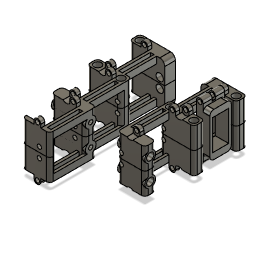
engine block (Autodesk Fusion 360 design; units mm, degrees)
Autodesk Fusion 360 part; units mm, degrees
note: some values were not read from the file. Chosen so that the rebuilt part matches the saved one: which face or edge a step refers to; which sketch regions a step uses.
sketch "Sketch1" plane through (0, 0, 0) normal (0, 1, 0) x (1, 0, 0)
  line L0 (0, 0) -> (2.7, 0)
  line L1 (2.7, 0) -> (2.7, -23.6)
  line L2 (2.7, -23.6) -> (0, -23.6)
  line L3 (0, -23.6) -> (0, 0)
  line L4 (-2, 2) -> (4.7, 2)
  line L5 (4.7, 2) -> (4.7, -25.6)
  line L6 (4.7, -25.6) -> (-2, -25.6)
  line L7 (-2, -25.6) -> (-2, 2)
  dimension "d1" = 2.7
  dimension "d2" = 23.6
  dimension "d3" = 2
  dimension "d4" = 2
  dimension "d5" = 2
  dimension "d6" = 2
  constraint horizontal L0
  constraint vertical L1
  constraint horizontal L2
  constraint vertical L3
  constraint coincident L0.start L3.end
  constraint horizontal L4
  constraint vertical L5
  constraint horizontal L6
  constraint vertical L7
  measures "d1" distance of L0.start L0.end
  measures "d2" distance of L0.start L2.end
  measures "d3" distance of L0 L4
  measures "d4" distance of L1 L5
  measures "d5" distance of L3 L7
  measures "d6" distance of L2 L6
extrude "Extrude1" add sketch "Sketch1" along normal blind 5 makes body 1
sketch "Sketch2" plane through (0, 5, 0) normal (0, 1, 0) x (-1, 0, 0)
  line L0 (-2.7, 23.6) -> (0, 23.6)
  line L1 (0, 23.6) -> (0, 0)
  line L2 (0, 0) -> (-2.7, 0)
  line L3 (-2.7, 0) -> (-2.7, 23.6)
  line L4 (2, 25.6) -> (-4.7, 25.6)
  line L5 (-4.7, 25.6) -> (-4.7, -2)
  line L6 (-4.7, -2) -> (2, -2)
  line L7 (2, -2) -> (2, 25.6)
  line L8 (2, -2) -> (-18.4, -2)
  line L9 (-18.4, -2) -> (-18.4, 0)
  line L10 (-18.4, 0) -> (2, 0)
  line L11 (2, 0) -> (2, -2)
  line L12 (2, 25.6) -> (-18.4, 25.6)
  line L13 (-18.4, 25.6) -> (-18.4, 23.6)
  line L14 (-18.4, 23.6) -> (2, 23.6)
  line L15 (2, 23.6) -> (2, 25.6)
  dimension "d9" = 20.4
  dimension "d10" = 20.4
  constraint horizontal L8
  constraint vertical L9
  constraint horizontal L10
  constraint vertical L11
  constraint coincident L6.end L7.start
  constraint coincident L1.end L10
  constraint horizontal L12
  constraint vertical L13
  constraint horizontal L14
  constraint vertical L15
  constraint coincident L4.start L7.end
  constraint coincident L0.end L14
  measures "d9" distance of L6.end L8.end
  measures "d10" distance of L4.start L12.end
extrude "Extrude2" add sketch "Sketch2" along normal blind 11.25 and the other way blind 5 contours L0 L4 L5 L7 L12 L14 L15 | L2 L5 L6 L7 L8 L10 L11 | L5 L12 L13 L14 | L5 L8 L9 L10 bodies 1
copy_body "CopyPasteBodies1" bodies 1 makes body 2
move_body "Move1" bodies 2 to x (1, 0, 0) y (0, 1, 0) z (0, 0, 1) at (-5, 0, 31.6)
extrude "Extrude3" add 1 faces at (-0.2, 5.4167, 29.6) along direction (0, 0, -1) blind 4 on bodies 2 bodies 2 1
extrude "Extrude4" add 1 faces at (-5.3333, 5.4167, 25.6) along direction (0, 0, -1) blind 2 on bodies 2 bodies 2
extrude "Extrude5" add 1 faces at (13.4, 5.4167, 27.6) along direction (1, 0, 0) blind 5 on bodies 2 bodies 2
sketch "Sketch3" plane through (0, 0, 0) normal (0, -1, 0) x (1, 0, 0)
  line L0 (2.7, 0) -> (0, 0)
  line L1 (0, 0) -> (0, 23.6)
  line L2 (0, 23.6) -> (2.7, 23.6)
  line L3 (2.7, 23.6) -> (2.7, 0)
  line L4 (-0.3, 31.6) -> (-0.3, 55.2)
  line L5 (-0.3, 55.2) -> (13.4, 55.2)
  line L6 (13.4, 55.2) -> (13.4, 57.2)
  line L7 (13.4, 57.2) -> (-7, 57.2)
  line L8 (-7, 57.2) -> (-7, 23.6)
  line L9 (-7, 23.6) -> (-2, 23.6)
  line L10 (-2, 23.6) -> (-2, -2)
  line L11 (-2, -2) -> (18.4, -2)
  line L12 (18.4, -2) -> (18.4, 0)
  line L13 (18.4, 0) -> (4.7, 0)
  line L14 (4.7, 0) -> (4.7, 23.6)
  line L15 (4.7, 23.6) -> (18.4, 23.6)
  line L16 (18.4, 23.6) -> (18.4, 31.6)
  line L17 (18.4, 31.6) -> (-0.3, 31.6)
  line L18 (-2.3, 31.6) -> (-5, 31.6)
  line L19 (-5, 31.6) -> (-5, 55.2)
  line L20 (-5, 55.2) -> (-2.3, 55.2)
  line L21 (-2.3, 55.2) -> (-2.3, 31.6)
  line L22 (-7, 23.6) -> (1, 23.6) construction
  line L23 (1, 23.6) -> (1, 31.6) construction
  line L24 (1, 31.6) -> (-7, 31.6) construction
  line L25 (-7, 31.6) -> (-7, 23.6) construction
  line L26 (-7, 31.6) -> (1, 23.6) construction
  circle A0 centre (-3, 27.6) radius 1.65
  circle A1 centre (-3, 27.6) radius 2.75
  line L27 (18.4, 31.6) -> (10.4, 31.6) construction
  line L28 (10.4, 31.6) -> (10.4, 23.6) construction
  line L29 (10.4, 23.6) -> (18.4, 23.6) construction
  line L30 (18.4, 23.6) -> (18.4, 31.6) construction
  line L31 (18.4, 31.6) -> (10.4, 23.6) construction
  circle A2 centre (14.4, 27.6) radius 1.65
  circle A3 centre (14.4, 27.6) radius 2.75
  dimension "d21" = 8
  dimension "d22" = 8
  dimension "d23" = 3.3
  dimension "d24" = 5.5
  dimension "d28" = 8
  dimension "d29" = 3.3
  dimension "d30" = 5.5
  constraint horizontal L22
  constraint vertical L23
  constraint horizontal L24
  constraint vertical L25
  constraint coincident L8.end L9.start
  constraint midpoint L26 A0.centre
  constraint concentric A0 A1
  constraint horizontal L27
  constraint vertical L28
  constraint horizontal L29
  constraint vertical L30
  constraint coincident L15 L28.end
  constraint coincident L16.end L17.start
  constraint midpoint L31 A2.centre
  constraint concentric A2 A3
  measures "d21" distance of L8.end L22.end
  measures "d22" distance of L8.end L24.end
  measures "d23" diameter of A0
  measures "d24" diameter of A1
  measures "d28" distance of L16.end L27.end
  measures "d29" diameter of A2
  measures "d30" diameter of A3
extrude "Extrude6" cut sketch "Sketch3" against normal through all contours A0 | A2 bodies 2
extrude "Extrude7" cut sketch "Sketch3" against normal blind 5 contours A1 | A3 bodies 2
fillet "Fillet1" radius 2.5 4 edges at (18.4, 8.125, 23.6) (18.4, 8.125, 31.6) (-7, 10.625, 31.6) (-7, 8.125, 23.6) on bodies 2
extrude "Extrude8" add 1 faces at (6.6, 5.4167, 57.2) along direction (0, 0, 1) blind 6 on bodies 2 bodies 2
fillet "Fillet2" radius 2.5 4 edges at (13.4, 8.125, 63.2) (13.4, 8.125, 55.2) (-7, 10.625, 55.2) (-7, 8.125, 63.2) on bodies 2
sketch "Sketch4" plane through (0, 0, 63.2) normal (0, 0, 1) x (1, 0, 0)
  line L0 (-4.5, 16.25) -> (-4.5, 0)
  line L1 (-4.5, 0) -> (10.9, 0)
  line L2 (10.9, 0) -> (10.9, 16.25)
  line L3 (10.9, 16.25) -> (-4.5, 16.25)
  line L4 (13.4, 0) -> (13.4, 16.25) construction
  line L5 (-0.3, 0) -> (13.4, 0) construction
  line L6 (-0.3, -5) -> (4.7, -5) construction
  line L7 (4.7, -5) -> (4.7, 0) construction
  line L8 (4.7, 0) -> (-0.3, 0) construction
  line L9 (-0.3, 0) -> (-0.3, -5) construction
  line L10 (4.7, 0) -> (-0.3, -5) construction
  arc A0 (-0.3, -2.5) -> (4.7, -2.5) centre (2.2, -2.5) ccw
  line L11 (-0.3, 0) -> (-0.3, -2.5)
  line L12 (4.7, -2.5) -> (4.7, 0)
  circle A1 centre (2.2, -2.5) radius 1.6
  point P0 (-0.3, 0)
  dimension "d38" = 5
  dimension "d39" = 5
  dimension "d40" = 3.2
  constraint coincident P0 L5.start
  constraint coincident L4.start L5.end
  constraint horizontal L6
  constraint vertical L7
  constraint horizontal L8
  constraint vertical L9
  constraint midpoint L7 A0.end
  constraint midpoint L9 A0.start
  constraint midpoint L10 A0.centre
  constraint concentric A0 A1
  measures "d38" distance of L6.start L6.end
  measures "d39" distance of L6.start P0
  measures "d40" diameter of A1
extrude "Extrude9" add sketch "Sketch4" against normal blind 3 from surface at -5 contours L1 A0 L11 L12 bodies 2
extrude "Extrude10" add sketch "Sketch4" against normal blind 3 from surface at -31.6 contours L1 A0 L11 L12 bodies 2
sketch "Sketch5" plane through (0, 0, 23.6) normal (0, 0, -1) x (-1, 0, 0)
  line L0 (4.5, 0) -> (4.5, 16.25)
  line L1 (4.5, 16.25) -> (-15.9, 16.25)
  line L2 (-15.9, 16.25) -> (-15.9, 0)
  line L3 (-15.9, 0) -> (-4.7, 0)
  line L4 (-4.7, 0) -> (-4.7, 5)
  line L5 (-4.7, 5) -> (-2.7, 5)
  line L6 (-2.7, 5) -> (-2.7, 0)
  line L7 (-2.7, 0) -> (0, 0)
  line L8 (0, 0) -> (0, 5)
  line L9 (0, 5) -> (2, 5)
  line L10 (2, 5) -> (2, 0)
  line L11 (2, 0) -> (4.5, 0)
  line L12 (-4.7, 0) -> (-9.7, 0) construction
  line L13 (-9.7, 0) -> (-9.7, -5) construction
  line L14 (-9.7, -5) -> (-4.7, -5) construction
  line L15 (-4.7, -5) -> (-4.7, 0) construction
  line L16 (-4.7, 0) -> (-9.7, -5) construction
  arc A0 (-9.7, -2.5) -> (-4.7, -2.5) centre (-7.2, -2.5) ccw
  line L17 (-9.7, 0) -> (-9.7, -2.5)
  line L18 (-4.7, -2.5) -> (-4.7, 0)
  circle A1 centre (-7.2, -2.5) radius 1.6
  dimension "d47" = 5
  dimension "d48" = 5
  dimension "d49" = 3.2
  constraint horizontal L12
  constraint vertical L13
  constraint horizontal L14
  constraint vertical L15
  constraint coincident L3.end L4.start
  constraint midpoint L15 A0.end
  constraint midpoint L16 A0.centre
  constraint tangent A0 L17
  constraint concentric A0 A1
  measures "d47" distance of L3.end L12.end
  measures "d48" distance of L3.end L14.end
  measures "d49" diameter of A1
extrude "Extrude11" add sketch "Sketch5" against normal blind 3 contours L3 A0 L17 L18 bodies 2
extrude "Extrude12" add sketch "Sketch5" along normal blind 3 from surface at 23.6 contours L3 A0 L17 L18 bodies 2
extrude "Extrude13" add 1 faces at (8.7, 10.8333, -2) along direction (0, 0, -1) blind 6 on bodies 2 bodies 2
fillet "Fillet3" radius 2.5 2 edges at (18.4, 8.125, 0) (18.4, 8.125, -8) on bodies 2
sketch "Sketch7" plane through (-2, 0, 0) normal (-1, 0, 0) x (0, 0, 1)
  line L0 (23.6, 0) -> (23.6, 5)
  line L1 (23.6, 5) -> (0, 5)
  line L2 (0, 5) -> (0, 16.25)
  line L3 (0, 16.25) -> (-8, 16.25)
  line L4 (-8, 16.25) -> (-8, 0)
  line L5 (-8, 0) -> (23.6, 0)
  line L6 (0, 5) -> (0, 0)
  constraint coincident L1.end L2.start
  constraint coincident L6.end origin
extrude "Extrude16" add sketch "Sketch7" along normal blind 6 contours L2 L3 L4 L5 L6 bodies 2
sketch "Sketch8" plane through (0, 0, 0) normal (0, 0, 1) x (1, 0, 0)
  line L0 (15.9, 0) -> (15.9, 16.25)
  line L1 (15.9, 16.25) -> (-8, 16.25)
  line L2 (-8, 16.25) -> (-8, 0)
  line L3 (-8, 0) -> (-2, 0)
  line L4 (-2, 0) -> (-2, 5)
  line L5 (-2, 5) -> (0, 5)
  line L6 (0, 5) -> (0, 0)
  line L7 (0, 0) -> (2.7, 0)
  line L8 (2.7, 0) -> (2.7, 5)
  line L9 (2.7, 5) -> (4.7, 5)
  line L10 (4.7, 5) -> (4.7, 0)
  line L11 (4.7, 0) -> (4.7, -2.5)
  arc A0 (4.7, -2.5) -> (9.7, -2.5) centre (7.2, -2.5) ccw
  line L12 (9.7, -2.5) -> (9.7, 0)
  line L13 (9.7, 0) -> (15.9, 0)
  circle A1 centre (7.2, -2.5) radius 1.6
  circle A2 centre (-4.25, 12.5) radius 3.75
  circle A3 centre (-4.25, 12.5) radius 2.75
  circle A4 centre (-4.25, 12.5) radius 1.6
  circle A5 centre (-4.25, 3.75) radius 3.75
  dimension "d69" = 5.5
  dimension "d70" = 1
  dimension "d71" = 3.2
  constraint tangent L2 A2
  constraint tangent L1 A2
  constraint concentric A2 A3
  constraint concentric A2 A4
  constraint tangent L3 A5
  constraint tangent L2 A5
  constraint equal A2 A5
  measures "d69" diameter of A3
  measures "d70" distance of A2 A3
  measures "d71" diameter of A4
extrude "Extrude17" cut sketch "Sketch8" against normal through all contours L2 L3 A5 | A4 bodies 2
extrude "Extrude18" cut sketch "Sketch8" against normal blind 4 contours A3 bodies 2
sketch "Sketch9" plane through (13.4, 0, 0) normal (1, 0, 0) x (0, 0, -1)
  line L0 (-57.7, 0) -> (-57.7, 16.25)
  line L1 (-57.7, 16.25) -> (-60.7, 16.25)
  line L2 (-60.7, 16.25) -> (-60.7, 0)
  line L3 (-60.7, 0) -> (-57.7, 0)
  line L4 (-60.7, 16.25) -> (-57.7, 0) construction
  circle A0 centre (-59.2, 8.125) radius 1.6
  line L5 (-55.2, 0) -> (-55.2, 16.25)
  line L6 (-63.2, 16.25) -> (-63.2, 0)
  circle A1 centre (-59.2, 8.125) radius 4
  circle A2 centre (-59.2, 8.125) radius 2.75
  dimension "d75" = 3.2
  dimension "d79" = 5.5
  constraint coincident L1.end L2.start
  constraint coincident L0.start L3.end
  constraint midpoint L4 A0.centre
  constraint concentric A0 A1
  constraint tangent L5 A1
  constraint concentric A0 A2
  measures "d75" diameter of A0
  measures "d79" diameter of A2
extrude "Extrude19" add sketch "Sketch9" against normal up to surface (20.4 mm away) contours L0 L2 A1 A2 | L0 A1 A2 | L0 L2 A0 A2 | L0 A0 A2 | L2 A1 A2 | L2 A0 A2 | L0 L2 A1 A2 | L0 L2 A0 A2 bodies 2
extrude "Extrude20" cut sketch "Sketch9" against normal through all contours L0 L2 A0 | L0 A0 | L2 A0 bodies 2
extrude "Extrude21" cut sketch "Sketch9" against normal blind 16 contours L0 L2 A0 A2 | L0 A0 A2 | L2 A0 A2 | L0 L2 A0 A2 bodies 2
extrude "Extrude22" cut sketch "Sketch8" along normal through all contours A4 bodies 2
sketch "Sketch20" plane through (0, 0, 0) normal (0, -1, 0) x (1, 0, 0)
  line L0 (-4.25, 0) -> (-4.25, -8)
  line L1 (-4.25, -8) -> (15.9, -8)
  arc A0 (15.9, -8) -> (18.4, -5.5) centre (15.9, -5.5) ccw
  line L2 (18.4, -5.5) -> (18.4, -2.5)
  arc A1 (18.4, -2.5) -> (15.9, 0) centre (15.9, -2.5) ccw
  line L3 (15.9, 0) -> (9.7, 0)
  line L4 (9.7, 0) -> (9.7, -3)
  line L5 (9.7, -3) -> (4.7, -3)
  line L6 (4.7, -3) -> (4.7, 0)
  line L7 (4.7, 0) -> (4.7, 23.6)
  line L8 (4.7, 23.6) -> (4.7, 26.6)
  line L9 (4.7, 26.6) -> (9.7, 26.6)
  line L10 (9.7, 26.6) -> (9.7, 23.6)
  line L11 (9.7, 23.6) -> (15.9, 23.6)
  arc A2 (15.9, 23.6) -> (18.4, 26.1) centre (15.9, 26.1) ccw
  line L12 (18.4, 26.1) -> (18.4, 29.1)
  arc A3 (18.4, 29.1) -> (15.9, 31.6) centre (15.9, 29.1) ccw
  line L13 (15.9, 31.6) -> (4.7, 31.6)
  line L14 (4.7, 31.6) -> (4.7, 28.6)
  line L15 (4.7, 28.6) -> (-0.3, 28.6)
  line L16 (-0.3, 28.6) -> (-0.3, 31.6)
  line L17 (-0.3, 31.6) -> (-0.3, 55.2)
  line L18 (-0.3, 55.2) -> (-0.3, 58.2)
  line L19 (-0.3, 58.2) -> (4.7, 58.2)
  line L20 (4.7, 58.2) -> (4.7, 55.2)
  line L21 (4.7, 55.2) -> (10.9, 55.2)
  arc A4 (10.9, 55.2) -> (13.4, 57.7) centre (10.9, 57.7) ccw
  line L22 (13.4, 57.7) -> (13.4, 60.7)
  arc A5 (13.4, 60.7) -> (10.9, 63.2) centre (10.9, 60.7) ccw
  line L23 (10.9, 63.2) -> (-4.5, 63.2)
  arc A6 (-4.5, 63.2) -> (-7, 60.7) centre (-4.5, 60.7) ccw
  line L24 (-7, 60.7) -> (-7, 26.1)
  arc A7 (-7, 26.1) -> (-4.5, 23.6) centre (-4.5, 26.1) ccw
  line L25 (-4.5, 23.6) -> (-2, 23.6)
  line L26 (-2, 23.6) -> (-2, 0)
  line L27 (-2, 0) -> (-4.25, 0)
  line L28 (2.7, 0) -> (0, 0)
  line L29 (0, 0) -> (0, 23.6)
  line L30 (0, 23.6) -> (2.7, 23.6)
  line L31 (2.7, 23.6) -> (2.7, 0)
  circle A8 centre (14.4, 27.6) radius 2.75
  circle A9 centre (-3, 27.6) radius 2.75
  line L32 (-5, 31.5495) -> (-5, 55.2505)
  arc A10 (-5, 55.2505) -> (-4.5, 55.2) centre (-4.5, 57.7) ccw
  line L33 (-4.5, 55.2) -> (-2.3, 55.2)
  line L34 (-2.3, 55.2) -> (-2.3, 31.6)
  line L35 (-2.3, 31.6) -> (-4.5, 31.6)
  arc A11 (-4.5, 31.6) -> (-5, 31.5495) centre (-4.5, 29.1) ccw
  circle A12 centre (14.4, -4) radius 4 construction
  circle A13 centre (14.4, -4) radius 1.6
  circle A14 centre (14.4, -4) radius 2.75
  dimension "d179" = 3.2
  dimension "d180" = 5.5
  constraint tangent L3 A12
  constraint tangent L2 A12
  constraint tangent L1 A12
  constraint concentric A12 A13
  constraint concentric A12 A14
  measures "d179" diameter of A13
  measures "d180" diameter of A14
extrude "Extrude41" cut sketch "Sketch20" against normal through all contours A13 bodies 2
extrude "Extrude42" cut sketch "Sketch20" against normal blind 5 contours A14 bodies 2
mirror "Mirror3" about plane through (-8, 0, 0) normal (-1, 0, 0) of bodies 2 makes body 3
move_body "Move2" bodies 3 to x (1, 0, 0) y (0, 1, 0) z (0, 0, 1) at (-20, 0, 0)
delete_face "DeleteFace1" 6 faces at (-30.7381, 4.7496, 63.0811) (-31.2766, 4.375, 55.21) (-30.4908, 8.3436, 55.206) (-31.2495, 9.2965, 55.2126) (-30.0678, 10.8018, 62.7491) (-30.1428, 7.2575, 63.1048) on bodies 3
sketch "Sketch12" plane through (0, 0, 0) normal (0, -1, 0) x (1, 0, 0)
  line L0 (-31, 55.2) -> (-31, 31.5495)
  arc A0 (-31, 31.5495) -> (-31.5, 31.6) centre (-31.5, 29.1) ccw
  line L1 (-31.5, 31.6) -> (-33.7, 31.6)
  line L2 (-33.7, 31.6) -> (-33.7, 55.2)
  line L3 (-33.7, 55.2) -> (-31, 55.2)
  circle A1 centre (-33, 27.6) radius 2.75
  circle A2 centre (-50.4, 27.6) radius 2.75
  line L4 (-36, 0) -> (-38.7, 0)
  line L5 (-38.7, 0) -> (-38.7, 23.6)
  line L6 (-38.7, 23.6) -> (-36, 23.6)
  line L7 (-36, 23.6) -> (-36, 0)
  line L8 (-29, 26.1) -> (-29, 63.2)
  line L9 (-29, 63.2) -> (-46.9, 63.2)
  arc A3 (-46.9, 63.2) -> (-49.4, 60.7) centre (-46.9, 60.7) ccw
  line L10 (-49.4, 60.7) -> (-49.4, 57.7)
  arc A4 (-49.4, 57.7) -> (-46.9, 55.2) centre (-46.9, 57.7) ccw
  line L11 (-46.9, 55.2) -> (-40.7, 55.2)
  line L12 (-40.7, 55.2) -> (-40.7, 58.2)
  line L13 (-40.7, 58.2) -> (-35.7, 58.2)
  line L14 (-35.7, 58.2) -> (-35.7, 55.2)
  line L15 (-35.7, 55.2) -> (-35.7, 31.6)
  line L16 (-35.7, 31.6) -> (-35.7, 28.6)
  line L17 (-35.7, 28.6) -> (-40.7, 28.6)
  line L18 (-40.7, 28.6) -> (-40.7, 31.6)
  line L19 (-40.7, 31.6) -> (-51.9, 31.6)
  arc A5 (-51.9, 31.6) -> (-54.4, 29.1) centre (-51.9, 29.1) ccw
  line L20 (-54.4, 29.1) -> (-54.4, 26.1)
  arc A6 (-54.4, 26.1) -> (-51.9, 23.6) centre (-51.9, 26.1) ccw
  line L21 (-51.9, 23.6) -> (-45.7, 23.6)
  line L22 (-45.7, 23.6) -> (-45.7, 26.6)
  line L23 (-45.7, 26.6) -> (-40.7, 26.6)
  line L24 (-40.7, 26.6) -> (-40.7, 23.6)
  line L25 (-40.7, 23.6) -> (-40.7, 0)
  line L26 (-40.7, 0) -> (-40.7, -3)
  line L27 (-40.7, -3) -> (-45.7, -3)
  line L28 (-45.7, -3) -> (-45.7, 0)
  line L29 (-45.7, 0) -> (-51.9, 0)
  arc A7 (-51.9, 0) -> (-54.4, -2.5) centre (-51.9, -2.5) ccw
  line L30 (-54.4, -2.5) -> (-54.4, -5.5)
  arc A8 (-54.4, -5.5) -> (-51.9, -8) centre (-51.9, -5.5) ccw
  line L31 (-51.9, -8) -> (-31.75, -8)
  line L32 (-31.75, -8) -> (-31.75, 0)
  line L33 (-31.75, 0) -> (-34, 0)
  line L34 (-34, 0) -> (-34, 23.6)
  line L35 (-34, 23.6) -> (-31.5, 23.6)
  arc A9 (-31.5, 23.6) -> (-29, 26.1) centre (-31.5, 26.1) ccw
  line L36 (-33.7, 55.2) -> (-33.7, 63.2) construction
  line L37 (-33.7, 63.2) -> (-28.7, 63.2) construction
  line L38 (-28.7, 63.2) -> (-26, 63.2)
  line L39 (-26, 63.2) -> (-26, 86.8)
  line L40 (-26, 86.8) -> (-28.7, 86.8)
  line L41 (-28.7, 86.8) -> (-28.7, 63.2)
  line L42 (-24, 88.8) -> (-30.7, 88.8)
  line L43 (-30.7, 88.8) -> (-30.7, 61.2)
  line L44 (-30.7, 61.2) -> (-24, 61.2) construction
  line L45 (-24, 61.2) -> (-24, 88.8)
  line L46 (-31, 55.2) -> (-24, 55.2)
  line L47 (-24, 55.2) -> (-24, 61.2)
  line L48 (-24, 61.2) -> (-31, 61.2)
  line L49 (-31, 61.2) -> (-31, 55.2) construction
  line L50 (-24, 86.8) -> (-44.4, 86.8) construction
  line L51 (-44.4, 86.8) -> (-44.4, 89.8)
  line L52 (-44.4, 89.8) -> (-24, 89.8)
  line L53 (-24, 89.8) -> (-24, 86.8)
  line L54 (-30.7, 86.8) -> (-44.4, 86.8)
  circle A10 centre (-50.4, -4) radius 2.75
  dimension "d107" = 5
  dimension "d108" = 2.7
  dimension "d109" = 23.6
  dimension "d110" = 2
  dimension "d111" = 2
  dimension "d112" = 2
  dimension "d113" = 2
  dimension "d114" = 20.4
  dimension "d115" = 3
  constraint coincident L2.end L3.start
  constraint coincident L9 L36.end
  constraint perpendicular L9 L36
  constraint perpendicular L36 L37
  constraint horizontal L38
  constraint vertical L39
  constraint horizontal L40
  constraint vertical L41
  constraint horizontal L42
  constraint vertical L43
  constraint horizontal L44
  constraint vertical L45
  constraint horizontal L46
  constraint vertical L47
  constraint horizontal L48
  constraint vertical L49
  constraint coincident L0.start L3.end
  constraint horizontal L50
  constraint vertical L51
  constraint horizontal L52
  constraint vertical L53
  constraint coincident L45 L50.start
  constraint coincident L39.end L50
  constraint coincident L50 L54.start
  constraint coincident L43 L54.start
  measures "d107" distance of L36.end L37.end
  measures "d108" distance of L37.end L38.end
  measures "d109" distance of L37.end L40.end
  measures "d110" distance of L40 L42
  measures "d111" distance of L39 L45
  measures "d112" distance of L41 L43
  measures "d113" distance of L38 L44
  measures "d114" distance of L50.start L50.end
  measures "d115" distance of L50.start L52.end
extrude "Extrude26" add sketch "Sketch12" against normal blind 5 contours L8 L9 L42 L43 L45 L48 L53 bodies 3
extrude "Extrude27" add sketch "Sketch12" against normal up to surface (16.25 mm away) contours L8 L46 L47 L48 | L42 L43 L51 L52 L53 L54 bodies 3
extrude "Extrude29" cut 1 faces at (-29, 8.5869, 59.1707) along direction (1, 0, 0) blind 5 on bodies 3 bodies 3
extrude "Extrude28" add 1 faces at (-29, 12.5, 61.8667) along direction (1, 0, 0) blind 5 on bodies 3 bodies 3
extrude "Extrude36" add 1 faces at (-26.2333, 8.75, 88.8) along direction (0, 0, -1) blind 2 on bodies 3 bodies 3
fillet "Fillet5" radius 2.5 4 edges at (-24, 10.625, 63.2) (-24, 8.125, 55.2) (-24, 8.125, 89.8) (-44.4, 8.125, 89.8) on bodies 3
extrude "Extrude30" add 1 faces at (-33.4, 6.016, 60.2599) along direction (-1, 0, 0) blind 2 from surface at -9.4 on bodies 3 bodies 3
extrude "Extrude31" add 1 faces at (-49.4, 2.9446, 59.7) along direction (-1, 0, 0) blind 7 from surface at -25.4 on bodies 3 bodies 3
sketch "Sketch13" plane through (0, 0, 63.2) normal (0, 0, 1) x (1, 0, 0)
  line L0 (-26.5, 8.125) -> (-26.5, 16.25)
  line L1 (-26.5, 16.25) -> (-46.9, 16.25)
  line L2 (-46.9, 16.25) -> (-46.9, 8.125)
  line L3 (-46.9, 8.125) -> (-46.9, 0)
  line L4 (-46.9, 0) -> (-30.7, 0)
  line L5 (-30.7, 0) -> (-30.7, 5)
  line L6 (-30.7, 5) -> (-28.7, 5)
  line L7 (-28.7, 5) -> (-28.7, 0)
  line L8 (-28.7, 0) -> (-26.5, 0)
  line L9 (-26.5, 0) -> (-26.5, 8.125)
  circle A0 centre (-31.75, 12.5) radius 1.6
extrude "Extrude32" cut sketch "Sketch13" along normal blind -8 and the other way blind -28 contours A0 bodies 3
sketch "Sketch14" plane through (0, 0, 63.2) normal (0, 0, 1) x (1, 0, 0)
  line L0 (-26.5, 8.125) -> (-26.5, 16.25)
  line L1 (-26.5, 16.25) -> (-46.9, 16.25)
  line L2 (-46.9, 16.25) -> (-46.9, 8.125)
  line L3 (-46.9, 8.125) -> (-46.9, 0)
  line L4 (-46.9, 0) -> (-30.7, 0)
  line L5 (-30.7, 0) -> (-30.7, 5)
  line L6 (-30.7, 5) -> (-28.7, 5)
  line L7 (-28.7, 5) -> (-28.7, 0)
  line L8 (-28.7, 0) -> (-26.5, 0)
  line L9 (-26.5, 0) -> (-26.5, 8.125)
  circle A0 centre (-31.75, 12.5) radius 1.6
  line L10 (-30.7, 0) -> (-35.7, 0) construction
  line L11 (-35.7, 0) -> (-35.7, -5) construction
  line L12 (-35.7, -5) -> (-30.7, -5) construction
  line L13 (-30.7, -5) -> (-30.7, 0) construction
  line L14 (-30.7, 0) -> (-35.7, -5) construction
  arc A1 (-35.7, -2.5) -> (-30.7, -2.5) centre (-33.2, -2.5) ccw
  line L15 (-35.7, -2.5) -> (-35.7, 0)
  line L16 (-30.7, 0) -> (-30.7, -2.5)
  circle A2 centre (-33.2, -2.5) radius 1.6
  dimension "d136" = 5
  dimension "d137" = 5
  dimension "d138" = 3.2
  constraint horizontal L10
  constraint vertical L11
  constraint horizontal L12
  constraint vertical L13
  constraint coincident L4.end L5.start
  constraint midpoint L13 A1.end
  constraint midpoint L14 A1.centre
  constraint tangent A1 L15
  constraint concentric A1 A2
  measures "d136" distance of L4.end L10.end
  measures "d137" distance of L4.end L12.end
  measures "d138" diameter of A2
extrude "Extrude33" add sketch "Sketch14" against normal blind 3 contours L4 A1 L15 L16 bodies 3
extrude "Extrude34" add sketch "Sketch14" along normal blind 3 from surface at 23.6 contours L4 A1 L15 L16 bodies 3
sketch "Sketch15" plane through (-49.4, 0, 0) normal (-1, 0, 0) x (0, 0, 1)
  circle A0 centre (59.2, 8.125) radius 2.75
  line L0 (60.7, 0) -> (60.7, 4.4169)
  arc A1 (60.7, 4.4169) -> (60.7, 11.8331) centre (59.2, 8.125) ccw
  line L1 (60.7, 11.8331) -> (60.7, 16.25)
  line L2 (60.7, 16.25) -> (57.7, 16.25)
  line L3 (57.7, 16.25) -> (57.7, 11.8331)
  arc A2 (57.7, 11.8331) -> (57.7, 4.4169) centre (59.2, 8.125) ccw
  line L4 (57.7, 4.4169) -> (57.7, 0)
  line L5 (57.7, 0) -> (60.7, 0)
  line L6 (57.4679, 11.125) -> (55.7359, 8.125)
  line L7 (55.7359, 8.125) -> (57.4679, 5.125)
  line L8 (57.4679, 5.125) -> (60.9321, 5.125)
  line L9 (60.9321, 5.125) -> (62.6641, 8.125)
  line L10 (62.6641, 8.125) -> (60.9321, 11.125)
  line L11 (60.9321, 11.125) -> (57.4679, 11.125)
  point P0 (59.2, 8.125)
  dimension "d144" = 3
  constraint coincident P0 A0.centre
  measures "d144" distance of P0 L11
extrude "Extrude35" cut sketch "Sketch15" against normal up to surface (16 mm away) contours L6 L7 L8 L9 L10 L11 bodies 3
sketch "Sketch16" plane through (0, 0, 26.6) normal (0, 0, 1) x (1, 0, 0)
  circle A0 centre (7.2, -2.5) radius 1.6
  line L0 (9.7, -2.5) -> (9.7, 0)
  line L1 (9.7, 0) -> (4.7, 0)
  line L2 (4.7, 0) -> (4.7, -2.5)
  arc A1 (4.7, -2.5) -> (9.7, -2.5) centre (7.2, -2.5) ccw
  circle A2 centre (7.2, -2.5) radius 3.5355
  constraint concentric A0 A2
  constraint coincident L0.end A2
extrude "Extrude37" cut sketch "Sketch16" along normal blind 5 contours L1 A2 bodies 2
sketch "Sketch17" plane through (0, 0, 58.2) normal (0, 0, 1) x (1, 0, 0)
  circle A0 centre (2.2, -2.5) radius 1.6
  line L0 (-0.3, 0) -> (-0.3, -2.5)
  arc A1 (-0.3, -2.5) -> (4.7, -2.5) centre (2.2, -2.5) ccw
  line L1 (4.7, -2.5) -> (4.7, 0)
  line L2 (4.7, 0) -> (-0.3, 0)
  circle A2 centre (2.2, -2.5) radius 3.3302
  constraint concentric A0 A2
  constraint coincident origin A2
extrude "Extrude38" cut sketch "Sketch17" along normal blind 5 contours L2 A2 bodies 2
sketch "Sketch18" plane through (0, 0, 26.6) normal (0, 0, 1) x (1, 0, 0)
  circle A0 centre (-43.2, -2.5) radius 1.6
  line L0 (-45.7, 0) -> (-45.7, -2.5)
  arc A1 (-45.7, -2.5) -> (-40.7, -2.5) centre (-43.2, -2.5) ccw
  line L1 (-40.7, -2.5) -> (-40.7, 0)
  line L2 (-40.7, 0) -> (-45.7, 0)
  circle A2 centre (-43.2, -2.5) radius 3.5355
  constraint concentric A0 A2
  constraint coincident L0.start A2
extrude "Extrude39" cut sketch "Sketch18" along normal blind 5 contours L2 A2 bodies 3
sketch "Sketch19" plane through (0, 0, 58.2) normal (0, 0, 1) x (1, 0, 0)
  circle A0 centre (-38.2, -2.5) radius 1.6
  line L0 (-35.7, -2.5) -> (-35.7, 0)
  line L1 (-35.7, 0) -> (-40.7, 0)
  line L2 (-40.7, 0) -> (-40.7, -2.5)
  arc A1 (-40.7, -2.5) -> (-35.7, -2.5) centre (-38.2, -2.5) ccw
  circle A2 centre (-38.2, -2.5) radius 3.5355
  constraint concentric A0 A2
  constraint coincident L1.end A2
extrude "Extrude40" cut sketch "Sketch19" along normal blind 5 contours L1 A2 bodies 3
mirror "Mirror1" about plane through (13.4, 16.25, 31.6) normal (0, 1, 0) of bodies 2 3 makes body 4 at (0.15, 32.5, -3.6667) makes body 5 at (-36.15, 32.5, -3.6667)
extrude "Extrude14" add 2 faces at (16.7731, 5, 27.4634) (-0.633, 5, 27.3814) along direction (0, -1, 0) blind 5 on bodies 2 bodies 2
sketch "Sketch6" plane through (0, 0, 0) normal (0, -1, 0) x (1, 0, 0)
  line L0 (-5, 31.5495) -> (-5, 55.2505)
  arc A0 (-5, 55.2505) -> (-4.5, 55.2) centre (-4.5, 57.7) ccw
  line L1 (-4.5, 55.2) -> (-2.3, 55.2)
  line L2 (-2.3, 55.2) -> (-2.3, 31.6)
  line L3 (-2.3, 31.6) -> (-4.5, 31.6)
  arc A1 (-4.5, 31.6) -> (-5, 31.5495) centre (-4.5, 29.1) ccw
  line L4 (0, 0) -> (0, 23.6)
  line L5 (0, 23.6) -> (2.7, 23.6)
  line L6 (2.7, 23.6) -> (2.7, 0)
  line L7 (-2, 0) -> (-4.25, 0)
  line L8 (-4.25, -8) -> (15.9, -8)
  arc A2 (15.9, -8) -> (18.4, -5.5) centre (15.9, -5.5) ccw
  line L9 (18.4, -5.5) -> (18.4, -2.5)
  arc A3 (18.4, -2.5) -> (15.9, 0) centre (15.9, -2.5) ccw
  line L10 (15.9, 0) -> (9.7, 0)
  line L11 (9.7, 0) -> (9.7, -3)
  line L12 (9.7, -3) -> (4.7, -3)
  line L13 (4.7, -3) -> (4.7, 0)
  line L14 (4.7, 0) -> (4.7, 23.6)
  line L15 (4.7, 23.6) -> (4.7, 26.6)
  line L16 (4.7, 28.6) -> (-0.3, 28.6)
  line L17 (-0.3, 28.6) -> (-0.3, 31.6)
  line L18 (-0.3, 31.6) -> (-0.3, 55.2)
  line L19 (-0.3, 55.2) -> (-0.3, 58.2)
  line L20 (-0.3, 58.2) -> (0, 58.2)
  line L21 (0, 63.2) -> (-4.5, 63.2)
  arc A4 (-4.5, 63.2) -> (-7, 60.7) centre (-4.5, 60.7) ccw
  line L22 (-7, 60.7) -> (-7, 26.1)
  arc A5 (-7, 26.1) -> (-4.5, 23.6) centre (-4.5, 26.1) ccw
  line L23 (-4.5, 23.6) -> (-2, 23.6)
  line L24 (-2, 23.6) -> (-2, 0)
  line L25 (-4.0402, 30.783) -> (-6.2766, 28.2907)
  line L26 (-6.2766, 28.2907) -> (-5.2365, 25.1077)
  line L27 (-5.2365, 25.1077) -> (-1.9598, 24.417)
  line L28 (-1.9598, 24.417) -> (0.2766, 26.9093)
  line L29 (0.2766, 26.9093) -> (-0.7635, 30.0923)
  line L30 (-0.7635, 30.0923) -> (-4.0402, 30.783)
  line L31 (12.7257, 30.5) -> (11.0514, 27.6)
  line L32 (11.0514, 27.6) -> (12.7257, 24.7)
  line L33 (12.7257, 24.7) -> (16.0743, 24.7)
  line L34 (16.0743, 24.7) -> (17.7486, 27.6)
  line L35 (17.7486, 27.6) -> (16.0743, 30.5)
  line L36 (16.0743, 30.5) -> (12.7257, 30.5)
  circle A6 centre (-3, 27.6) radius 1.65
  line L37 (-4.25, 0) -> (-4.25, -8)
  line L38 (2.7, 0) -> (0, 0)
  line L39 (-31, 55.2) -> (-31, 31.5495)
  arc A7 (-31, 31.5495) -> (-31.5, 31.6) centre (-31.5, 29.1) ccw
  line L40 (-31.5, 31.6) -> (-33.7, 31.6)
  line L41 (-33.7, 31.6) -> (-33.7, 55.2)
  line L42 (-33.7, 55.2) -> (-31, 55.2)
  line L43 (-36, 0) -> (-38.7, 0)
  line L44 (-38.7, 0) -> (-38.7, 23.6)
  line L45 (-38.7, 23.6) -> (-36, 23.6)
  line L46 (-36, 23.6) -> (-36, 0)
  circle A8 centre (-33, 27.6) radius 2.75
  line L47 (-26, 86.8) -> (-26, 63.1495)
  arc A9 (-26, 63.1495) -> (-26.5, 63.2) centre (-26.5, 60.7) ccw
  line L48 (-26.5, 63.2) -> (-28.7, 63.2)
  line L49 (-28.7, 63.2) -> (-28.7, 86.8)
  line L50 (-28.7, 86.8) -> (-26, 86.8)
  line L51 (-30.7, 89.8) -> (-30.7, 86.8)
  line L52 (-30.7, 86.8) -> (-30.7, 63.2)
  line L53 (-30.7, 63.2) -> (-30.7, 60.2)
  line L54 (-30.7, 60.2) -> (-35.7, 60.2)
  line L55 (-35.7, 58.2) -> (-35.7, 55.2)
  line L56 (-35.7, 55.2) -> (-35.7, 31.6)
  line L57 (-35.7, 31.6) -> (-35.7, 28.6)
  line L58 (-35.7, 28.6) -> (-40.7, 28.6)
  line L59 (-40.7, 26.6) -> (-40.7, 23.6)
  line L60 (-40.7, 23.6) -> (-40.7, 0)
  line L61 (-40.7, 0) -> (-40.7, -3)
  line L62 (-40.7, -3) -> (-45.7, -3)
  line L63 (-45.7, -3) -> (-45.7, 0)
  line L64 (-45.7, 0) -> (-51.9, 0)
  arc A10 (-51.9, 0) -> (-54.4, -2.5) centre (-51.9, -2.5) ccw
  line L65 (-54.4, -2.5) -> (-54.4, -5.5)
  arc A11 (-54.4, -5.5) -> (-51.9, -8) centre (-51.9, -5.5) ccw
  line L66 (-51.9, -8) -> (-31.75, -8)
  line L67 (-31.75, -8) -> (-31.75, 0)
  line L68 (-31.75, 0) -> (-34, 0)
  line L69 (-34, 0) -> (-34, 23.6)
  line L70 (-34, 23.6) -> (-31.5, 23.6)
  arc A12 (-31.5, 23.6) -> (-29, 26.1) centre (-31.5, 26.1) ccw
  line L71 (-29, 26.1) -> (-29, 55.2)
  line L72 (-29, 55.2) -> (-26.5, 55.2)
  arc A13 (-26.5, 55.2) -> (-24, 57.7) centre (-26.5, 57.7) ccw
  line L73 (-24, 57.7) -> (-24, 87.3)
  arc A14 (-24, 87.3) -> (-26.5, 89.8) centre (-26.5, 87.3) ccw
  line L74 (-26.5, 89.8) -> (-30.7, 89.8)
  line L75 (-35.3282, 30.0068) -> (-36.2485, 26.7871)
  line L76 (-36.2485, 26.7871) -> (-33.9203, 24.3803)
  line L77 (-33.9203, 24.3803) -> (-30.6718, 25.1932)
  line L78 (-30.6718, 25.1932) -> (-29.7515, 28.4129)
  line L79 (-29.7515, 28.4129) -> (-32.0797, 30.8197)
  line L80 (-32.0797, 30.8197) -> (-35.3282, 30.0068)
  line L81 (-48.0726, 30.0076) -> (-51.3214, 30.8194)
  line L82 (-51.3214, 30.8194) -> (-53.6487, 28.4118)
  line L83 (-53.6487, 28.4118) -> (-52.7274, 25.1924)
  line L84 (-52.7274, 25.1924) -> (-49.4786, 24.3806)
  line L85 (-49.4786, 24.3806) -> (-47.1513, 26.7882)
  line L86 (-47.1513, 26.7882) -> (-48.0726, 30.0076)
  line L87 (0, 58.2) -> (0, 63.2)
  line L88 (4.7, 26.6) -> (4.7, 28.6)
  line L89 (-35.7, 60.2) -> (-35.7, 58.2)
  line L90 (-40.7, 28.6) -> (-40.7, 26.6)
  circle A15 centre (14.4, -4) radius 2.75
  circle A16 centre (-50.4, -4) radius 2.75
  line L91 (17.3, -2.3257) -> (14.4, -0.6514)
  line L92 (14.4, -0.6514) -> (11.5, -2.3257)
  line L93 (11.5, -2.3257) -> (11.5, -5.6743)
  line L94 (11.5, -5.6743) -> (14.4, -7.3486)
  line L95 (14.4, -7.3486) -> (17.3, -5.6743)
  line L96 (17.3, -5.6743) -> (17.3, -2.3257)
  line L97 (-47.5, -2.3257) -> (-50.4, -0.6514)
  line L98 (-50.4, -0.6514) -> (-53.3, -2.3257)
  line L99 (-53.3, -2.3257) -> (-53.3, -5.6743)
  line L100 (-53.3, -5.6743) -> (-50.4, -7.3486)
  line L101 (-50.4, -7.3486) -> (-47.5, -5.6743)
  line L102 (-47.5, -5.6743) -> (-47.5, -2.3257)
  point P0 (-3, 27.6)
  point P1 (14.4, 27.6)
  point P2 (-33, 27.6)
  point P3 (-50.4, 27.6)
  point P4 (14.4, -4)
  point P5 (-50.4, -4)
  dimension "d61" = 2.9
  dimension "d62" = 2.9
  dimension "d169" = 2.9
  dimension "d170" = 2.9
  dimension "d184" = 2.9
  dimension "d185" = 2.9
  constraint coincident P0 A6.centre
  constraint coincident P2 A8.centre
  constraint coincident P4 A15.centre
  constraint coincident P5 A16.centre
  measures "d61" distance of P0 L30
  measures "d62" distance of P1 L36
  measures "d169" distance of P2 L80
  measures "d170" distance of P3 L86
  measures "d184" distance of P4 L96
  measures "d185" distance of P5 L102
extrude "Extrude15" cut sketch "Sketch6" against normal blind 5 contours L16 L17 L29 | L16 L17 L25 L26 L27 L28 L29 L30 | L31 L32 L33 L34 L35 L36 | L57 L58 L75 L76 L77 L78 L79 L80 | L81 L82 L83 L84 L85 L86 | L91 L92 L93 L94 L95 L96 | L97 L98 L99 L100 L101 L102 bodies 2 3
sketch "Sketch10" plane through (0, 0, 0) normal (1, 0, 0) x (0, 0, -1)
  line L0 (-14, 27.6) -> (-2, 27.6)
  line L1 (-2, 27.6) -> (-2, 4.9)
  line L2 (-2, 4.9) -> (-14, 4.9)
  line L3 (-14, 4.9) -> (-14, 27.6)
  line L4 (-16, 32.5) -> (0, 32.5)
  line L5 (0, 32.5) -> (0, 0)
  line L6 (0, 0) -> (-16, 0)
  line L7 (-16, 0) -> (-16, 32.5)
  line L8 (-8, 27.6) -> (-8, 32.5) construction
  line L9 (-8, 4.9) -> (-8, 0) construction
  dimension "d83" = 12
  dimension "d84" = 22.7
  dimension "d86" = 2
  dimension "d87" = 2
  dimension "d89" = 32.5
  constraint horizontal L0
  constraint vertical L1
  constraint horizontal L2
  constraint vertical L3
  constraint horizontal L4
  constraint vertical L5
  constraint horizontal L6
  constraint vertical L7
  constraint midpoint L0 L8.start
  constraint midpoint L4 L8.end
  constraint midpoint L2 L9.start
  constraint midpoint L6 L9.end
  constraint equal L8 L9
  constraint coincident L5.end L6.start
  measures "d83" distance of L0.start L0.end
  measures "d84" distance of L0.start L2.end
  measures "d86" distance of L3 L7
  measures "d87" distance of L1 L5
  measures "d89" distance of L4.end L5.end
extrude "Extrude23" add sketch "Sketch10" along normal blind 10 separate body makes body 6
sketch "Sketch11" plane through (0, 0, 16) normal (0, 0, 1) x (1, 0, 0)
  line L0 (0, 32.5) -> (0, 0)
  line L1 (0, 0) -> (10, 0)
  line L2 (10, 0) -> (10, 32.5)
  line L3 (10, 32.5) -> (0, 32.5)
  line L4 (0, 32.5) -> (5, 32.5) construction
  line L5 (5, 32.5) -> (5, 37.5)
  line L6 (5, 37.5) -> (0, 37.5) construction
  line L7 (0, 37.5) -> (0, 32.5)
  line L8 (0, 32.5) -> (5, 37.5) construction
  arc A0 (5, 35) -> (0, 35) centre (2.5, 35) ccw
  circle A1 centre (2.5, 35) radius 1.6
  line L9 (4.1743, 37.9) -> (0.8257, 37.9)
  line L10 (0.8257, 37.9) -> (-0.8486, 35)
  line L11 (-0.8486, 35) -> (0.8257, 32.1)
  line L12 (0.8257, 32.1) -> (4.1743, 32.1)
  line L13 (4.1743, 32.1) -> (5.8486, 35)
  line L14 (5.8486, 35) -> (4.1743, 37.9)
  point P0 (2.5, 35)
  dimension "d92" = 5
  dimension "d93" = 5
  dimension "d94" = 3.2
  dimension "d95" = 2.9
  constraint horizontal L4
  constraint vertical L5
  constraint horizontal L6
  constraint vertical L7
  constraint coincident L0.start L3.end
  constraint midpoint L7 A0.end
  constraint midpoint L5 A0.start
  constraint midpoint L8 P0
  constraint concentric A0 A1
  constraint coincident P0 A0.centre
  constraint parallel L4 L12
  measures "d92" distance of L0.start L4.end
  measures "d93" distance of L0.start L6.end
  measures "d94" diameter of A1
  measures "d95" distance of P0 L14
extrude "Extrude24" add sketch "Sketch11" against normal blind 16 contours L3 L7 L11 | L3 L5 L7 A0 L11 L13 | L3 L5 L13 bodies 6
extrude "Extrude25" cut sketch "Sketch11" along normal mid plane 2.5 from surface at -8 contours L3 L5 L7 A0 L11 L13 | L3 L11 L12 L13 bodies 6
ref_plane "WorkPlane1" through (5, 16.25, 8) normal (0, 1, 0) x (0, 0, 1)
mirror "Mirror2" about plane through (5, 16.25, 8) normal (0, 1, 0) of "Extrude24", "Extrude25"
fillet "Fillet4" radius 3 4 edges at (7.5, 32.5, 16) (7.5, 32.5, 0) (7.5, 0, 16) (7.5, 0, 0) on bodies 6
copy_body "Body->Comp1" bodies 2 removing the originals makes body 7 in component "short bottom"
copy_body "Body->Comp2" bodies 3 removing the originals makes body 8 in component "long bottom"
copy_body "Body->Comp3" bodies 4 removing the originals makes body 9 in component "short top"
copy_body "Body->Comp4" bodies 5 removing the originals makes body 10 in component "long top"
copy_body "Body->Comp5" bodies 6 removing the originals makes body 11 in component "motor slider"
component "short bottom" placed x (1, 0, 0) y (0, 1, 0) z (0, 0, 1) at (0, 0, 0)
component "long bottom" placed x (1, 0, 0) y (0, 1, 0) z (0, 0, 1) at (-7, 0, 0)
component "short top" placed x (1, 0, 0) y (0, 1, 0) z (0, 0, 1) at (0, 0, 0)
component "long top" placed x (1, 0, 0) y (0, 1, 0) z (0, 0, 1) at (-7, 0, 0)
component "motor slider" placed x (1, 0, 0) y (0, 1, 0) z (0, 0, 1) at (4.7, 0, 0)
equation "d2 = ( 11.8 * 2 ) * 1 mm"
named bodies: "short bottom", "short top", "motor slider", "long bottom", "long top"
